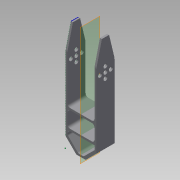
# Autodesk Inventor part: Leg
Saved by Autodesk Inventor 2014 (Build 180170000, 170)
## iProperties
Created: 2014-03-07
Part Number: Leg
Material: Générique
Document SubType Name: Modeling
Designer: Grégoire
Density: 1 g/cm^3
Appearance: Par défaut
Author: Grégoire
Autodesk Inventor part; units mm, degrees
ref_plane "YZ Plane" through (0, 0, 0) normal (1, 0, 0) x (0, 1, 0)
ref_plane "XZ Plane" through (0, 0, 0) normal (0, 1, 0) x (-1, 0, 0)
ref_plane "XY Plane" through (0, 0, 0) normal (0, 0, 1) x (1, 0, 0)
sketch "Esquisse1" plane through (0, 0, 0) normal (0, 0, 1) x (1, 0, 0)
  line L0 (0, 0) -> (34.4, 0)
  line L1 (34.4, 0) -> (34.4, 20)
  line L2 (34.4, 20) -> (0, 20)
  line L3 (0, 20) -> (0, 0)
  dimension "d0" = 34.4
  dimension "d1" = 20
  constraints: 8 end point, 2 parallel, 1 horizontal, 1 perpendicular
  measures "d0" distance of L1.end L2.end
  measures "d1" distance of L0.end L1.end
extrude "Extrusion1" add sketch "Esquisse1" along normal blind 2.2
sketch "Esquisse2" plane through (0, 0, 2.2) normal (0, 0, 1) x (1, 0, 0)
  line L0 (0, 0) -> (34.4, 0) projected
  line L1 (34.4, 20) -> (0, 20) projected
  line L2 (0, 20) -> (0, 0) projected
  line L3 (0, 20) -> (2.2, 20)
  line L4 (2.2, 20) -> (2.2, 0)
  line L5 (2.2, 0) -> (0, 0)
  line L6 (0, 0) -> (0, 20)
  line L7 (17.2, 20) -> (17.2, 0) construction
  line L8 (34.4, 20) -> (32.2, 20)
  line L9 (32.2, 20) -> (32.2, 0)
  line L10 (32.2, 0) -> (34.4, 0)
  line L11 (34.4, 0) -> (34.4, 20)
  dimension "d4" = 2.2
  constraints: 18 end point, 3 symmetric about line, 2 midpoint, 2 parallel, 1 horizontal, 1 perpendicular, 1 point on line
  measures "d4" distance between parallel lines of L4 L2
extrude "Extrusion2" add sketch "Esquisse2" along normal blind 92 contours L2 L1 L4 L0 | L9 L1 L11 L0
sketch "Esquisse3" plane through (34.4, 0, 0) normal (1, 0, 0) x (0, 0, -1)
  line L0 (0, 0) -> (0, 20) construction
  line L1 (-94.2, 0) -> (-94.2, 20) construction
  line L2 (-94.2, 10) -> (0, 10) construction
  circle A0 centre (-85.2, 10) radius 2.21
  line L3 (-85.2, 10) -> (-85.2, 15.2246) construction
  circle A1 centre (-79.2, 10) radius 2.21
  circle A2 centre (-91.2, 10) radius 2.21
  circle A3 centre (-85.2, 10) radius 2.21
  circle A4 centre (-85.2, 16) radius 2.21
  circle A5 centre (-85.2, 4) radius 2.21
  circle A6 centre (-85.2, 10) radius 2.21
  dimension "d7" = 9
  dimension "d8" = 4.42
  dimension "d11" = 6
  dimension "d14" = 6
  dimension "d19" = 6
  dimension "d22" = 6
  constraints: 7 centre point, 4 end point, 2 horizontal, 2 midpoint, 2 vertical, 1 perpendicular, 1 point on line, 12 other
  measures "d7" distance of L2.start L3.start
  measures "d8" diameter of A0
  measures "d11" distance of L3.start A1.centre
  measures "d14" distance of L3.start A2.centre
  measures "d19" distance of L3.start A4.centre
  measures "d22" distance of L3.start A5.centre
extrude "Extrusion3" cut sketch "Esquisse3" against normal through all
chamfer "Chanfrein1" distance 12 angle 45 4 edges at (2.2, 10, 2.2) (32.2, 10, 2.2) (0, 10, 0) (34.4, 10, 0)
sketch "Esquisse6" plane through (12, 20, 0) normal (0, 1, 0) x (1, 0, 0)
  line L0 (-9.8, -14.2) -> (-9.8, -94.2) construction
  line L1 (20.2, -14.2) -> (20.2, -94.2) construction
  line L2 (22.4, -86.2) -> (20.2, -86.2) construction
  line L3 (-9.8, -41.2) -> (20.2, -41.2)
  line L4 (20.2, -41.2) -> (20.2, -39)
  line L5 (20.2, -39) -> (-9.8, -39)
  line L6 (-9.8, -39) -> (-9.8, -41.2)
  line L7 (-9.8, -21.2) -> (20.2, -21.2)
  line L8 (20.2, -21.2) -> (20.2, -19)
  line L9 (20.2, -19) -> (-9.8, -19)
  line L10 (-9.8, -19) -> (-9.8, -21.2)
  point P0 (-9.8, -86.2)
  dimension "d43" = 45
  dimension "d44" = 2.2
  dimension "d50" = 20
  constraints: 16 end point, 2 parallel, 2 point on line, 1 horizontal, 1 perpendicular, 1 vertical, 8 other
  measures "d43" distance between parallel lines of L2 L3
  measures "d44" distance between parallel lines of L5 L3
  measures "d50" distance of L4.end L9.start
extrude "Extrusion5" add sketch "Esquisse6" against normal blind 20
fillet "Congé3" radius 3 10 edges at (32.2, 10, 41.2) (2.2, 10, 41.2) (2.2, 10, 39) (2.2, 10, 19) (32.2, 10, 39) (32.2, 10, 21.2) (2.2, 10, 21.2) (2.2, 10, 14.2) (14.2, 10, 2.2) (20.2, 10, 2.2)
sketch "Esquisse7" plane through (0, 0, 94.2) normal (-1, 0, 0) x (0, 0, 1)
  line L0 (-82.2, 0) -> (0, 0) construction
  line L1 (0, 20) -> (0, 0) construction
  line L2 (-82.2, 20) -> (0, 20) construction
  line L3 (0, 20) -> (25, 14)
  line L4 (25, 14) -> (25, 6)
  line L5 (25, 6) -> (0, 0)
  line L6 (0, 20) -> (0, 0)
  line L7 (25, 10) -> (0, 10) construction
  point P0 (-94.2, 0)
  dimension "d55" = 8
  dimension "d56" = 25
  constraints: 10 end point, 3 perpendicular, 2 midpoint
  measures "d55" distance of L3.end L4.end
  measures "d56" horizontal distance of L1.start L3.end
extrude "Extrusion6" add sketch "Esquisse7" against normal blind 2.2
ref_plane "Plan de construction2" through (17.2, 0, 12) normal (-1, 0, 0) x (0, 0, 1)
mirror "Symétrie1" about plane through (17.2, 0, 12) normal (-1, 0, 0) of "Extrusion6"
fillet "Congé4" radius 10 4 edges at (1.1, 20, 94.2) (1.1, 0, 94.2) (33.3, 0, 94.2) (33.3, 20, 94.2)
sketch "Esquisse8" plane through (0, 0, 12) normal (-1, 0, 0) x (0, 0, 1)
  arc A0 (81.0168, 0) -> (83.3505, 0.2761) centre (81.0168, 10) ccw construction
  line L0 (83.3505, 0.2761) -> (107.2, 6) construction
  line L1 (107.2, 6) -> (107.2, 14) construction
  line L2 (107.2, 14) -> (83.3505, 19.7239) construction
  arc A1 (83.3505, 19.7239) -> (81.0168, 20) centre (81.0168, 10) ccw construction
  line L3 (0, 20) -> (81.0168, 20) construction
  line L4 (0, 0) -> (0, 20) construction
  line L5 (0, 0) -> (81.0168, 0) construction
  circle A2 centre (73.2, 4) radius 2.21 construction
  circle A3 centre (79.2, 10) radius 2.21 construction
  circle A4 centre (73.2, 10) radius 2.21 construction
  circle A5 centre (67.2, 10) radius 2.21 construction
  circle A6 centre (73.2, 16) radius 2.21 construction
  line L6 (107.2, 14) -> (90.5333, 10)
  line L7 (90.5333, 10) -> (107.2, 6)
  line L8 (107.2, 14) -> (107.2, 6)
  line L9 (90.5333, 10) -> (107.2, 10) construction
  point P0 (-12, 0)
  constraints: 8 end point, 2 perpendicular, 1 midpoint, 1 parallel
equation "\"d2\" = UDepth"
equation "\"d4\" = Depth"
equation "\"d8\" = Holes"
equation "\"d44\" = Depth"
equation "\"d57\" = Depth"
equation "\"Depth\" = 2.2"
equation "\"Holes\" = 4.42"
equation "\"UDepth\" = Depth"
equation "\"URound\" = 8"
